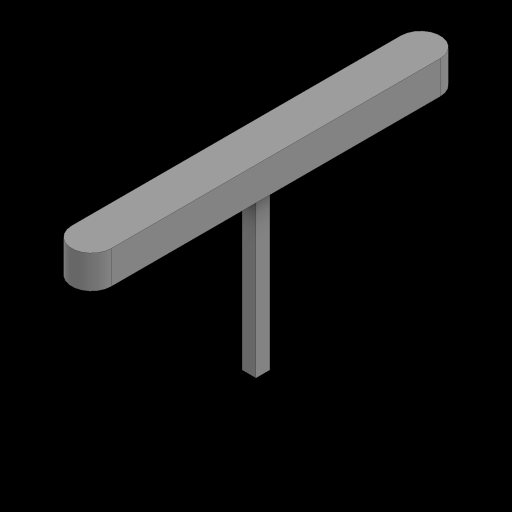
# Autodesk Inventor part: rp_lever
Saved by Autodesk Inventor 2023 (Build 270158000, 158)
## iProperties
Created: 2024-07-04
Part Number: rp_lever
Material: 일반
Document SubType Name: Modeling
Designer: OMS55
Density: 1 g/cm^3
Appearance: 기본값
Mass: 8.64051 g
Surface Area: 37.7708 cm^2
Volume: 8.64051 cm^3
Author: OMS55
Autodesk Inventor part; units mm, degrees
ref_plane "YZ Plane" through (0, 0, 0) normal (1, 0, 0) x (0, 1, 0)
ref_plane "XZ Plane" through (0, 0, 0) normal (0, 1, 0) x (-1, 0, 0)
ref_plane "XY Plane" through (0, 0, 0) normal (0, 0, 1) x (1, 0, 0)
sketch "스케치1" plane through (0, 0, 0) normal (0, 1, 0) x (-1, 0, 0)
  circle A0 centre (0, 0) radius 3.1
  line L0 (2.1, 2.1) -> (-2.1, 2.1)
  line L1 (-2.1, 2.1) -> (-2.1, -2.1)
  line L2 (-2.1, -2.1) -> (2.1, -2.1)
  line L3 (2.1, -2.1) -> (2.1, 2.1)
  point P0 (2.1, 0)
  point P1 (0, 2.1)
  dimension "d0" = 6.2
  dimension "d7" = 4.2
  dimension "d8" = 4.2
  constraints: 8 end point, 2 midpoint, 1 centre point, 1 coincident, 1 horizontal, 1 horizontal alignment, 1 parallel, 1 perpendicular, 1 vertical alignment
  measures "d0" diameter of A0
  measures "d7" distance of L0.start L0.end
  measures "d8" distance of L0.end L1.end
extrude "돌출1" add sketch "스케치1" along normal blind 50 contours L3 L2 L1 L0
sketch "스케치2" plane through (0, 50, 0) normal (0, 1, 0) x (1, 0, 0)
  line L0 (0, -50) -> (0, 50) construction
  line L1 (6, -50) -> (6, 50)
  line L2 (-6, 50) -> (-6, -50)
  arc A0 (-6, -50) -> (6, -50) centre (0, -50) ccw
  arc A1 (6, 50) -> (-6, 50) centre (0, 50) ccw
  point P0 (0, 0)
  point P1 (0, 0)
  point P2 (-6, 0)
  dimension "d3" = 100
  dimension "d4" = 6
  constraints: 8 end point, 4 point on circle, 4 tangent, 2 centre point, 2 midpoint, 1 coincident, 1 horizontal alignment, 1 parallel, 1 vertical
  measures "d3" distance of L2.start L2.end
  measures "d4" radius of A1
extrude "돌출2" add sketch "스케치2" along normal blind 10
